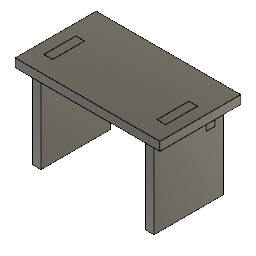
TestcutCNC v6 (Autodesk Fusion 360 design; units mm, degrees)
Autodesk Fusion 360 part; units mm, degrees
sketch "TableLegSketch" plane through (0, 0, 0) normal (1, 0, 0) x (0, 1, 0)
  line L0 (0, 0) -> (10, 0)
  line L1 (10, 0) -> (10, 140)
  line L2 (10, 140) -> (0, 140)
  line L3 (0, 140) -> (0, 0)
  line L4 (130, 140) -> (130, 0)
  line L5 (130, 0) -> (10, 0)
  line L6 (10, 0) -> (10, 140)
  line L7 (130, 140) -> (140, 140)
  line L8 (140, 140) -> (140, 0)
  line L9 (140, 0) -> (130, 0)
  line L10 (130, 0) -> (130, 140)
  line L11 (100, 140) -> (100, 110)
  line L12 (100, 110) -> (115, 110)
  line L13 (115, 110) -> (115, 140)
  line L14 (115, 140) -> (130, 140)
  line L15 (30, 140) -> (30, 155)
  line L16 (30, 155) -> (85, 155)
  line L17 (85, 155) -> (85, 140)
  line L18 (10, 140) -> (30, 140)
  line L19 (85, 140) -> (100, 140)
  dimension "d3" = 10
  dimension "d4" = 140
  constraint horizontal L0
  constraint vertical L1
  constraint horizontal L2
  constraint vertical L3
  constraint coincident L0.start L3.end
  constraint horizontal L18
  constraint vertical L4
  constraint horizontal L5
  constraint vertical L6
  constraint horizontal L7
  constraint vertical L8
  constraint horizontal L9
  constraint vertical L10
  constraint vertical L11
  constraint horizontal L12
  constraint vertical L13
  constraint coincident L13.end L18
  constraint collinear L14 L18
  constraint vertical L15
  constraint horizontal L16
  constraint vertical L17
  constraint coincident L17.end L18
  constraint collinear L18 L19
  measures "d3" distance of L0.start L0.end
  measures "d4" distance of L0.start L2.end
extrude "Extrude1" add sketch "TableLegSketch" along normal blind 15 from surface at 20 contours L1 L4 L5 L6 L10 L11 L12 L13 L14 L15 L16 L17 L18 L19 makes body 1
extrude "Extrude2" add 1 faces at (35, 80, 36.6667) along direction (1, 0, 0) blind 15 from surface at 180 on bodies 1 bodies 1 makes body 2
sketch "TableTop" plane through (0, 0, 0) normal (0, 0, 1) x (1, 0, 0)
  line L0 (0, 0) -> (250, 0)
  line L1 (250, 0) -> (250, 140)
  line L2 (250, 140) -> (0, 140)
  line L3 (0, 140) -> (0, 0)
  dimension "d11" = 250
  dimension "d12" = 140
  constraint horizontal L0
  constraint vertical L1
  constraint horizontal L2
  constraint vertical L3
  constraint coincident L0.start L3.end
  measures "d11" distance of L0.start L0.end
  measures "d12" distance of L0.start L2.end
extrude "Extrude3" add sketch "TableTop" along normal blind 15 from surface at 140 separate body makes body 3
sketch "MiddleSupportSketch" plane through (0, 115, 0) normal (0, -1, 0) x (1, 0, 0)
  line L0 (20, 140) -> (20, 110)
  line L1 (20, 110) -> (35, 110)
  line L2 (35, 110) -> (35, 140)
  line L3 (35, 140) -> (20, 140)
  line L4 (230, 110) -> (230, 140)
  line L5 (230, 140) -> (20, 140)
  line L6 (20, 140) -> (20, 110)
  line L7 (215, 110) -> (215, 85)
  line L8 (215, 85) -> (35, 85)
  line L9 (35, 85) -> (35, 110)
  line L10 (20, 110) -> (35, 110)
  line L11 (215, 110) -> (230, 110)
  constraint horizontal L10
  constraint vertical L4
  constraint horizontal L5
  constraint vertical L6
  constraint coincident L0.end L1.start
  constraint vertical L7
  constraint horizontal L8
  constraint vertical L9
  constraint coincident L1.end L2.start
  constraint collinear L10 L11
extrude "Extrude4" add sketch "MiddleSupportSketch" along normal blind 15 separate body makes body 4
combine "Combine1" operation cut target body 3 tool bodies 1 keep tools
combine "Combine2" operation cut target body 3 tool bodies 2 keep tools
sketch "TABLETOP" plane through (0, 0, 155) normal (0, 0, 1) x (-1, 0, 0)
  line L0 (-215, -85) -> (-230, -85)
  line L1 (-230, -85) -> (-230, -30)
  line L2 (-230, -30) -> (-215, -30)
  line L3 (-215, -30) -> (-215, -85)
  line L4 (-20, -85) -> (-35, -85)
  line L5 (-35, -85) -> (-35, -30)
  line L6 (-35, -30) -> (-20, -30)
  line L7 (-20, -30) -> (-20, -85)
  line L8 (0, -140) -> (0, 0)
  line L9 (0, 0) -> (-250, 0)
  line L10 (-250, 0) -> (-250, -140)
  line L11 (-250, -140) -> (0, -140)
sketch "LEGS" plane through (35, 0, 0) normal (1, 0, 0) x (0, 1, 0)
  line L0 (130, 0) -> (130, 140)
  line L1 (130, 140) -> (115, 140)
  line L2 (115, 140) -> (115, 110)
  line L3 (115, 110) -> (100, 110)
  line L4 (100, 110) -> (100, 140)
  line L5 (100, 140) -> (85, 140)
  line L6 (85, 140) -> (85, 155)
  line L7 (85, 155) -> (30, 155)
  line L8 (30, 155) -> (30, 140)
  line L9 (30, 140) -> (10, 140)
  line L10 (10, 140) -> (10, 0)
  line L11 (10, 0) -> (130, 0)
sketch "MIDDLESUPPORT" plane through (0, 100, 0) normal (0, -1, 0) x (1, 0, 0)
  line L0 (215, 85) -> (215, 110)
  line L1 (215, 110) -> (230, 110)
  line L2 (230, 110) -> (230, 140)
  line L3 (230, 140) -> (20, 140)
  line L4 (20, 140) -> (20, 110)
  line L5 (20, 110) -> (35, 110)
  line L6 (35, 110) -> (35, 85)
  line L7 (35, 85) -> (215, 85)
